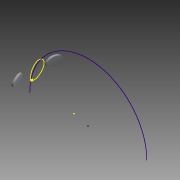
# Autodesk Inventor part: GhostIrisi
Saved by Autodesk Inventor 2015 (Build 190159000, 159)
## iProperties
Created: 2015-04-11
Part Number: GhostIrisi
Material: Generic
Document SubType Name: Modeling
Designer: tquinn
Density: 1 g/cm^3
Appearance: Default
Author: tquinn
Autodesk Inventor part; units mm, degrees
ref_plane "YZ Plane" through (0, 0, 0) normal (1, 0, 0) x (0, 1, 0)
ref_plane "XZ Plane" through (0, 0, 0) normal (0, 1, 0) x (-1, 0, 0)
ref_plane "XY Plane" through (0, 0, 0) normal (0, 0, 1) x (1, 0, 0)
sketch "Sketch1" plane through (0, 0, 0) normal (0, 0, 1) x (1, 0, 0)
  arc A0 (15.7789, -0.7835) -> (-9.6211, -0.7835) centre (3.0789, -0.7835) ccw
  spline S0 degree 3 poles (-9.1745, 1.7565) (-9.0723, 1.7565) (-8.9373, 1.8236) (-8.63, 2.0798) (-8.4577, 2.2685) (-8.1133, 2.7045) (-7.9142, 2.9901) (-7.5231, 3.6209) (-7.3311, 3.966) (-7.0154, 4.6029) (-6.8667, 4.9394) (-6.6393, 5.5737) (-6.5613, 5.8715) (-6.5035, 6.3359) (-6.5169, 6.5286) (-6.6312, 6.7787) (-6.7314, 6.8365) (-6.975, 6.8365) (-7.1386, 6.7682) (-7.4932, 6.5076) (-7.6841, 6.3151) (-8.0407, 5.8773) (-8.2339, 5.5973) (-8.5975, 4.9726) (-8.7679, 4.628) (-9.0388, 3.9886) (-9.1606, 3.651) (-9.3412, 3.0185) (-9.4002, 2.7237) (-9.4452, 2.2635) (-9.436, 2.0696) (-9.3485, 1.8162) (-9.2701, 1.7565) (-9.1745, 1.7565) knots 0 0 0 0 0.103206 0.103206 0.206413 0.206413 0.317066 0.317066 0.427718 0.427718 0.530317 0.530317 0.632916 0.632916 0.730045 0.730045 0.827173 0.827173 0.933966 0.933966 1.040759 1.040759 1.148764 1.148764 1.256768 1.256768 1.357087 1.357087 1.457406 1.457406 1.554012 1.554012 1.650618 1.650618 1.650618 1.650618 projected
  point P0 (0, 0)
  point P1 (-9.1745, 1.7565)
  constraints: 2 point on circle, 1 centre point, 4 other
sketch "Sketch2" plane through (0, 0, 0) normal (1, 0, 0) x (0, 1, 0)
  spline S0 degree 3 poles (1.7565, -3.81) (1.7565, -3.5032) (1.816, -3.168) (2.069, -2.5437) (2.2628, -2.2547) (2.7236, -1.7877) (3.0191, -1.5881) (3.652, -1.3295) (3.9893, -1.27) (4.6288, -1.27) (4.9736, -1.3386) (5.5979, -1.6026) (5.8774, -1.7977) (6.3145, -2.237) (6.5069, -2.5144) (6.7679, -3.1342) (6.8365, -3.4766) (6.8365, -4.1107) (6.7793, -4.4424) (6.5301, -5.065) (6.3376, -5.3558) (5.8718, -5.8318) (5.5729, -6.0326) (4.938, -6.2914) (4.6019, -6.35) (3.9654, -6.35) (3.62, -6.2822) (2.9885, -6.0142) (2.7025, -5.8139) (2.2675, -5.3672) (2.0795, -5.0934) (1.8238, -4.4794) (1.7565, -4.139) (1.7565, -3.81) knots 0 0 0 0 0.096675 0.096675 0.193351 0.193351 0.293983 0.293983 0.394615 0.394615 0.503491 0.503491 0.612368 0.612368 0.720266 0.720266 0.828164 0.828164 0.925474 0.925474 1.022784 1.022784 1.126104 1.126104 1.229423 1.229423 1.341412 1.341412 1.453401 1.453401 1.557082 1.557082 1.660763 1.660763 1.660763 1.660763 projected
  spline S1 degree 3 poles (1.7565, 3.81) (1.7565, 4.139) (1.8238, 4.4794) (2.0795, 5.0934) (2.2675, 5.3672) (2.7025, 5.8139) (2.9885, 6.0142) (3.62, 6.2822) (3.9654, 6.35) (4.6019, 6.35) (4.938, 6.2914) (5.5729, 6.0326) (5.8718, 5.8318) (6.3376, 5.3558) (6.5301, 5.065) (6.7793, 4.4424) (6.8365, 4.1107) (6.8365, 3.4766) (6.7679, 3.1342) (6.5069, 2.5144) (6.3145, 2.237) (5.8774, 1.7977) (5.5979, 1.6026) (4.9736, 1.3386) (4.6288, 1.27) (3.9893, 1.27) (3.652, 1.3295) (3.0191, 1.5881) (2.7236, 1.7877) (2.2628, 2.2547) (2.069, 2.5437) (1.816, 3.168) (1.7565, 3.5032) (1.7565, 3.81) knots 0 0 0 0 0.103681 0.103681 0.207362 0.207362 0.319351 0.319351 0.431339 0.431339 0.534659 0.534659 0.637979 0.637979 0.735288 0.735288 0.832598 0.832598 0.940496 0.940496 1.048394 1.048394 1.157271 1.157271 1.266148 1.266148 1.36678 1.36678 1.467412 1.467412 1.564087 1.564087 1.660763 1.660763 1.660763 1.660763 projected
  line L0 (6.8365, 3.81) -> (1.7565, 3.81)
  line L1 (6.8365, -3.81) -> (1.7565, -3.81)
  line L2 (4.2706, 6.3499) -> (4.2706, -6.3499)
  circle A0 centre (3.3816, 3.175) radius 1.27
  circle A1 centre (3.3816, -4.445) radius 1.27
  point P0 (0, 0)
  dimension "d0" = 2.54
  dimension "d1" = 2.54
  dimension "d2" = 0.635
  dimension "d3" = 0.635
  dimension "d4" = 0.889
  dimension "d5" = 0.889
  constraints: 6 end point, 2 centre point, 1 horizontal, 1 parallel, 1 perpendicular, 4 other
  measures "d0" diameter of A0
  measures "d1" diameter of A1
  measures "d2" distance from line of L0 A0.centre
  measures "d3" distance from line of L1 A1.centre
  measures "d4" distance from line of L2 A0.centre
  measures "d5" distance from line of A1.centre L2
extrude "Extrusion1" add sketch "Sketch2" against normal blind 25.4 contours A1 L2 L1 | L1 L2 A1 | A1 L1 L2 | L2 L1 A1 | A0 L0 L2 | L2 L0 A0 | L0 L2 A0 | A0 L2 L0
sketch "Sketch3" plane through (0, 0, 0) normal (0, 0, 1) x (1, 0, 0)
  arc A0 (15.7789, -0.7835) -> (-9.6211, -0.7835) centre (3.0789, -0.7835) ccw projected
  spline S0 degree 3 poles (-9.1745, 1.7565) (-9.0723, 1.7565) (-8.9373, 1.8236) (-8.63, 2.0798) (-8.4577, 2.2685) (-8.1133, 2.7045) (-7.9142, 2.9901) (-7.5231, 3.6209) (-7.3311, 3.966) (-7.0154, 4.6029) (-6.8667, 4.9394) (-6.6393, 5.5737) (-6.5613, 5.8715) (-6.5035, 6.3359) (-6.5169, 6.5286) (-6.6312, 6.7787) (-6.7314, 6.8365) (-6.975, 6.8365) (-7.1386, 6.7682) (-7.4932, 6.5076) (-7.6841, 6.3151) (-8.0407, 5.8773) (-8.2339, 5.5973) (-8.5975, 4.9726) (-8.7679, 4.628) (-9.0388, 3.9886) (-9.1606, 3.651) (-9.3412, 3.0185) (-9.4002, 2.7237) (-9.4452, 2.2635) (-9.436, 2.0696) (-9.3485, 1.8162) (-9.2701, 1.7565) (-9.1745, 1.7565) knots 0 0 0 0 0.103206 0.103206 0.206413 0.206413 0.317066 0.317066 0.427718 0.427718 0.530317 0.530317 0.632916 0.632916 0.730045 0.730045 0.827173 0.827173 0.933966 0.933966 1.040759 1.040759 1.148764 1.148764 1.256768 1.256768 1.357087 1.357087 1.457406 1.457406 1.554012 1.554012 1.650618 1.650618 1.650618 1.650618 projected
  circle A1 centre (3.0789, -0.7835) radius 13.589
  line L0 (3.0789, -0.7835) -> (3.0789, 12.8055)
  line L1 (3.0789, -0.7835) -> (-10.5101, -0.7835)
  line L2 (-10.5101, -0.7835) -> (-9.6211, -0.7835)
  line L3 (3.0789, 11.9165) -> (3.0789, 12.8055)
  arc A2 (3.0789, 12.8055) -> (-10.5101, -0.7835) centre (3.0789, -0.7835) ccw
  arc A3 (3.0789, 11.9165) -> (-9.6211, -0.7835) centre (3.0789, -0.7835) ccw
  circle A4 centre (3.0789, -0.7835) radius 13.208
  line L4 (3.0789, 12.8055) -> (3.0789, 12.4245)
  line L5 (-10.5101, -0.7835) -> (-10.1291, -0.7835)
  point P0 (0, 0)
  point P1 (-9.1745, 1.7565)
  dimension "d8" = 0.889
  dimension "d10" = 0.508
  constraints: 12 end point, 10 point on circle, 4 centre point, 3 concentric, 3 point on line, 2 coincident, 2 collinear, 1 perpendicular, 1 vertical
  measures "d8" radial gap between concentric circles of A0 A1
  measures "d10" radial gap between concentric circles of A0 A4
revolve "Revolution1" cut sketch "Sketch3" angle 360 about axis through (3.0789, -0.7835, 0) along (0, 1, 0) keep common part picked at (-1.8046, 11.6804) contours A4 L1 A1 L0
equation "\"d3\" = d2"
equation "\"d5\" = d4"
body "Solid1"
